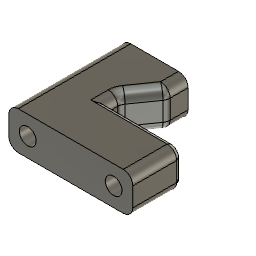
Altendorf_F-45_Stopper (Autodesk Fusion 360 design; units mm, degrees)
Autodesk Fusion 360 part; units mm, degrees
sketch "Sketch1" plane through (0, 0, 0) normal (0, 1, 0) x (1, 0, 0)
  line L0 (0, 0) -> (45, 0) construction
  circle A0 centre (45, 0) radius 6.75
  circle A1 centre (0, 0) radius 6.75
  circle A2 centre (0, 0) radius 4.4
  circle A3 centre (45, 0) radius 4.4
  line L1 (-10, -10) -> (55, -10)
  line L2 (55, -10) -> (55, 10)
  line L3 (55, 10) -> (-10, 10)
  line L4 (-10, 10) -> (-10, -10)
  line L5 (22.5, -10) -> (22.5, 10) construction
  dimension "d1" = 45
  dimension "d2" = 8.8
  dimension "d3" = 13.5
  dimension "d4" = 20
  dimension "d5" = 65
  constraint coincident L0.start A1.centre
  constraint horizontal L0
  constraint coincident L0.end A0.centre
  constraint equal A2 A3
  constraint equal A0 A1
  constraint horizontal L1
  constraint vertical L2
  constraint horizontal L3
  constraint vertical L4
  constraint midpoint L1 L5.start
  constraint midpoint L3 L5.end
  constraint midpoint L0 L5
  measures "d1" distance of L0.start L0.end
  measures "d2" diameter of A3
  measures "d3" diameter of A0
  measures "d4" distance of L1.end L2.end
  measures "d5" distance of L2.end L3.end
sketch "Sketch2" plane through (0, 0, 0) normal (0, 0, 1) x (1, 0, 0)
  line L0 (55, 0) -> (-10, 0)
  line L1 (-10, 0) -> (-10, -60)
  line L2 (-10, -60) -> (55, -60)
  line L3 (55, -60) -> (55, 0)
  line L4 (15, -35) -> (55, -35)
  line L5 (15, -35) -> (15, -26.2815)
  line L6 (15, -26.2815) -> (25, -12)
  line L7 (25, -12) -> (25, 0)
  line L8 (0, 0) -> (45, 0)
  dimension "d6" = 60
  dimension "d7" = 10
  dimension "d8" = 25
  dimension "d9" = 25
  dimension "d10" = 145
  dimension "d11" = 12
  constraint coincident L0.end L1.start
  constraint perpendicular L0 L1
  constraint perpendicular L1 L2
  constraint coincident L0.start L3.end
  constraint perpendicular L0 L3
  constraint coincident L3 L4.end
  constraint perpendicular L3 L4
  constraint perpendicular L4 L5
  constraint perpendicular L0 L7
  constraint coincident L7.end L8
  measures "d6" distance of L2.end L0.start
  measures "d7" distance of L5 L7
  measures "d8" distance of L2 L4
  measures "d9" distance of L1 L5
  measures "d10" angle of L5 L6
  measures "d11" distance of L6.end L7.end
extrude "Extrude1" add sketch "Sketch2" along normal up to surface (10 mm away) and the other way up to surface (10 mm away) contours L0 L1 L2 L3 L4 L5 L6 L7 L8
fillet "Fillet1" radius 5 12 edges at (25, -6, 10) (25, -6, -10) (-10, -30, -10) (-10, -30, 10) (55, -47.5, -10) (55, -47.5, 10) (20, -19.1407, 10) (20, -19.1407, -10) (25, -12, 0) (15, -30.6407, 10) (15, -30.6407, -10) (15, -26.2815, 0)
extrude "Extrude2" cut sketch "Sketch1" against normal through all contours A2 | A3
extrude "Extrude3" cut sketch "Sketch1" against normal blind 8 contours A1
extrude "Extrude4" cut sketch "Sketch1" against normal blind 8 from surface at -35 contours A0
chamfer "Chamfer1" distance 1 distance2 2 13 edges at (-10, 0, 0) (-8.5355, 0, -8.5355) (7.5, 0, -10) (23.5355, 0, -8.5355) (25, 0, 0) (23.5355, 0, 8.5355) (7.5, 0, 10) (-8.5355, 0, 8.5355) (30, -35, 10) (53.5355, -35, 8.5355) (55, -35, 0) (53.5355, -35, -8.5355) (30, -35, -10) measured on face at (-10, -20, -1.6667) measured on face at (-5.2379, -20, -9.9943) measured on face at (18.9167, 0, 0) measured on face at (24.9943, -6.949, -5.2379) measured on face at (25, -3.4745, -1.6667) measured on face at (24.9943, -6.949, 5.2379) measured on face at (18.9167, 0, 0) measured on face at (-9.9774, -40, 5.4753) measured on face at (22.75, -35, 0) measured on face at (50.2379, -51.6667, 9.9943) measured on face at (55, -51.6667, -1.6667) measured on face at (50.2379, -51.6667, -9.9943) measured on face at (22.75, -35, 0)
equation "d8 = 33 mm - 8 mm"
